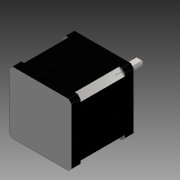
# Autodesk Inventor part: 步进电机
Saved by Autodesk Inventor 2016 (Build 200138000, 138)
## iProperties
Created: 2019-05-19
Part Number: 步进电机
Material: 常规
Document SubType Name: Modeling
Designer: oldboy
Density: 1 g/cm^3
Appearance: 默认
Author: oldboy
Autodesk Inventor part; units mm, degrees
sketch "草图1" plane through (0, 0, 0) normal (0, 1, 0) x (-1, 0, 0)
  line L0 (-21, 21) -> (21, 21)
  line L1 (21, 21) -> (21, -21)
  line L2 (21, -21) -> (-21, -21)
  line L3 (-21, -21) -> (-21, 21)
  line L4 (-21, 21) -> (21, -21) construction
  line L5 (21, 21) -> (-21, -21) construction
  point P0 (0, 0)
  dimension "d0" = 42
  constraints: 12 end point, 2 midpoint, 2 parallel, 2 perpendicular, 1 horizontal
  measures "d0" distance between parallel lines of L3 L1
extrude "拉伸1" add sketch "草图1" along normal blind 42
sketch "草图2" plane through (0, 42, 0) normal (0, 1, 0) x (1, 0, 0)
  circle A0 centre (0, 0) radius 15
  circle A1 centre (0, 0) radius 12.5
  dimension "d3" = 30
  dimension "d4" = 25
  constraints: 2 centre point, 2 coincident
  measures "d3" diameter of A0
  measures "d4" diameter of A1
extrude "拉伸2" cut sketch "草图2" against normal blind 1
sketch "草图3" plane through (0, 42, 0) normal (0, 1, 0) x (1, 0, 0)
  circle A0 centre (-18, -18) radius 1.5
  line L0 (0, 29.4) -> (0, -29.4) construction
  line L1 (-29.4, 0) -> (29.4, 0) construction
  circle A1 centre (18, -18) radius 1.5
  line L2 (29.4, 0) -> (-29.4, 0) construction
  circle A2 centre (-18, 18) radius 1.5
  circle A3 centre (18, 18) radius 1.5
  point P0 (0, 0)
  dimension "d8" = 3
  dimension "d9" = 18
  dimension "d10" = 18
  constraints: 5 symmetric about line, 4 centre point, 2 end point, 3 other
  measures "d8" diameter of A0
  measures "d9" distance from line of L0 A0.centre
  measures "d10" distance from line of L1 A0.centre
hole "孔1" at (18, 42, 18) at (-18, 42, 18) at (-18, 42, -18) at (18, 42, -18) direction (0, -1, 0) diameter 3 depth 10 tip angle 118
thread "螺纹1" size "M3x0.5" class "6H" standard "ANSI Metric M Profile" full length
thread "螺纹2" size "M3x0.5" class "6H" standard "ANSI Metric M Profile" full length
thread "螺纹3" size "M3x0.5" class "6H" standard "ANSI Metric M Profile" full length
thread "螺纹4" size "M3x0.5" class "6H" standard "ANSI Metric M Profile" full length
ref_plane "工作平面2" through (0, 42, 0) normal (0, 1, 0) x (1, 0, 0)
sketch "草图4" plane through (0, 42, 0) normal (0, 1, 0) x (1, 0, 0)
  circle A0 centre (0, 0) radius 2.5
  dimension "d26" = 5
  constraints: 1 centre point, 1 coincident
  measures "d26" diameter of A0
extrude "拉伸3" add sketch "草图4" along normal blind 25
ref_plane "工作平面3" through (0, 67, 0) normal (0, 1, 0) x (1, 0, 0)
sketch "草图5" plane through (0, 67, 0) normal (0, 1, 0) x (1, 0, 0)
  circle A0 centre (0, 0) radius 2.5 projected
  line L0 (-2, -1.5) -> (2, -1.5)
  dimension "d29" = 1.5
  constraints: 2 end point, 2 point on circle, 1 horizontal
  measures "d29" distance from line of point (0, 0) L0
extrude "拉伸4" cut sketch "草图5" against normal blind 15 contours L0 A0 picked at (-0.533956, -1.639793)
ref_plane "工作平面1" through (0, 21, 0) normal (0, 1, 0) x (1, 0, 0)
sketch "草图6" plane through (0, 21, 0) normal (0, 1, 0) x (1, 0, 0)
  circle A0 centre (-18, -18) radius 1.5
  line L0 (0, 29.4) -> (0, -29.4) construction
  line L1 (29.4, 0) -> (-29.4, 0) construction
  line L2 (-21, 21) -> (-21, -21)
  line L3 (-21, -21) -> (21, -21)
  line L4 (21, -21) -> (21, 21)
  line L5 (21, 21) -> (-21, 21)
  line L6 (-17.12132, -21) -> (-21, -17.12132)
  line L7 (-17.12132, 21) -> (-21, 17.12132)
  line L8 (17.12132, -21) -> (21, -17.12132)
  line L9 (17.12132, 21) -> (21, 17.12132)
  point P0 (0, 0)
  dimension "d34" = 45
  constraints: 8 end point, 6 symmetric about line, 2 point on line, 1 tangent
  measures "d34" angle of L3 L6
sketch "草图6 outline for 拉伸5" plane through (0, 21, 0) normal (0, 1, 0) x (1, 0, 0)
  line L0 (-21, -17.12132) -> (-21, -21)
  line L1 (-17.12132, -21) -> (-21, -17.12132)
  line L2 (-21, -21) -> (-17.12132, -21)
extrude "拉伸5" cut sketch "草图6 outline for 拉伸5" along normal mid plane 30
mirror "镜像1" about plane through (0, 0, 0) normal (1, 0, 0) of "拉伸5"
mirror "镜像2" about plane through (0, 0, 0) normal (0, 0, 1) of "拉伸5", "镜像1"
chamfer "倒角1" distance 2 angle 45 8 edges at (21, 39, -21) (21, 3, -21) (-21, 3, -21) (-21, 39, -21) (21, 39, 21) (21, 3, 21) (-21, 39, 21) (-21, 3, 21)
sketch "草图7" plane through (0, 42, 0) normal (0, 1, 0) x (1, 0, 0)
  circle A0 centre (0, 0) radius 2.5 projected
  circle A1 centre (0, 0) radius 12.5 projected
extrude "拉伸6" add sketch "草图7" along normal blind 1
fillet "圆角2" radius 0.5 1 edges at (-12.5, 43, 0)
